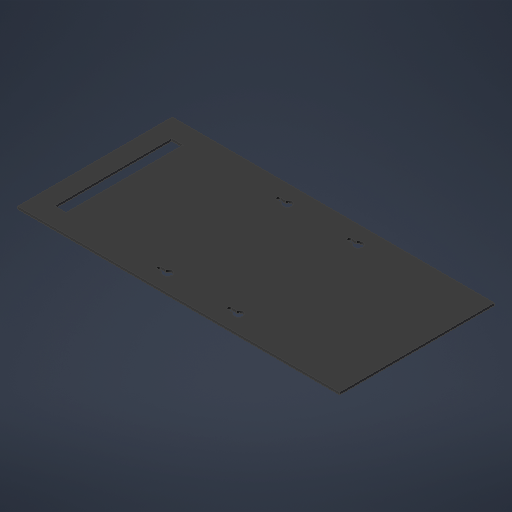
# Autodesk Inventor part: CoverImpresoraTermica
Saved by Autodesk Inventor 2026.1 (Build 301233020, 233B)
## iProperties
Created: 2025-11-04
Part Number: CoverImpresoraTermica
Material: Generic
Document SubType Name: Modeling
Designer: Tito Luyo Murata
Density: 1 g/cm^3
Appearance: Default
Author: Tito Luyo Murata
Autodesk Inventor part; units mm, degrees
ref_plane "YZ Plane" through (0, 0, 0) normal (1, 0, 0) x (0, 1, 0)
ref_plane "XZ Plane" through (0, 0, 0) normal (0, 1, 0) x (-1, 0, 0)
ref_plane "XY Plane" through (0, 0, 0) normal (0, 0, 1) x (1, 0, 0)
sketch "Sketch1" plane through (0, 0, 0) normal (0, 1, 0) x (-1, 0, 0)
  line L0 (0, 0) -> (250, 0)
  line L1 (250, 0) -> (250, -120)
  line L2 (250, -120) -> (0, -120)
  line L3 (0, -120) -> (0, 0)
  arc A0 (95.1623, -105) -> (95.1623, -108) centre (92, -106.5) ccw
  line L4 (236, -14.5) -> (227, -14.5)
  line L5 (227, -14.5) -> (227, -105.5)
  line L6 (227, -105.5) -> (236, -105.5)
  line L7 (236, -105.5) -> (236, -14.5)
  line L8 (95.1623, -105) -> (99, -105)
  line L9 (99, -108) -> (95.1623, -108)
  arc A1 (99, -108) -> (99, -105) centre (99, -106.5) ccw
  arc A2 (99, -15) -> (99, -12) centre (99, -13.5) ccw
  line L10 (95.1623, -12) -> (99, -12)
  arc A3 (95.1623, -12) -> (95.1623, -15) centre (92, -13.5) ccw
  line L11 (99, -15) -> (95.1623, -15)
  arc A4 (154, -108) -> (154, -105) centre (154, -106.5) ccw
  line L12 (150.1623, -105) -> (154, -105)
  arc A5 (150.1623, -105) -> (150.1623, -108) centre (147, -106.5) ccw
  line L13 (154, -108) -> (150.1623, -108)
  arc A6 (154, -15) -> (154, -12) centre (154, -13.5) ccw
  line L14 (150.1623, -12) -> (154, -12)
  arc A7 (150.1623, -12) -> (150.1623, -15) centre (147, -13.5) ccw
  line L15 (154, -15) -> (150.1623, -15)
  point P0 (0, -60)
  point P1 (250, -60)
  dimension "d0" = 250
  dimension "d1" = 120
  dimension "d4" = 7
  dimension "d5" = 92
  dimension "d14" = 9
  dimension "d15" = 91
  dimension "d16" = 45.5
  dimension "d28" = 46.5
  dimension "d31" = 3
  dimension "d32" = 7
  dimension "d33" = 1.5
  dimension "d34" = 3
  dimension "d35" = 7
  dimension "d38" = 93
  dimension "d41" = 55
  dimension "d44" = 80
  constraints: 32 end point, 16 point on circle, 8 centre point, 5 parallel, 4 horizontal, 2 midpoint, 2 perpendicular, 1 vertical, 30 other
  measures "d0" distance of L1.end L2.end
  measures "d1" distance of L0.end L1.end
  measures "d4" diameter of A0
  measures "d5" distance from line of L3 A0.centre
  measures "d14" distance between parallel lines of L5 L7
  measures "d15" distance between parallel lines of L6 L4
  measures "d16" distance from line of point (250, -60) L4
  measures "d28" vertical distance of point (0, -60) A0.centre
  measures "d31" distance between parallel lines of L9 L8
  measures "d32" horizontal distance of A0.centre L8.end
  measures "d33" vertical distance of A0.centre L8.end
  measures "d34" diameter of A1
  measures "d35" distance of A0.centre A1.centre
  measures "d38" distance of A1.centre A2.centre
  measures "d41" distance of A1.centre A4.centre
  measures "d44" distance from line of A5.centre L5
extrude "Extrusion1" add sketch "Sketch1" along normal blind 2
equation "\"d4\" = hueco_diam"
equation "\"d5\" = primer_hueco_dist"
equation "\"d14\" = boca_alto"
equation "\"d15\" = boca_ancho"
equation "\"d16\" = 0.5 * boca_ancho"
equation "\"d28\" = 0.5 * huecos_horiz_dist"
equation "\"d31\" = hueco_ranura_ancho"
equation "\"d32\" = -0.5 * hueco_diam + hueco_ranura_largo - 0.5 * hueco_ranura_ancho"
equation "\"d33\" = 0.5 * hueco_ranura_ancho"
equation "\"d34\" = hueco_ranura_ancho"
equation "\"d35\" = -0.5 * hueco_diam + hueco_ranura_largo - 0.5 * hueco_ranura_ancho"
equation "\"d38\" = huecos_horiz_dist"
equation "\"d41\" = hueco_vertical_dist"
equation "\"d44\" = boca_vertical_dist"
equation "\"hueco_diam\" = 7"
equation "\"primer_hueco_dist\" = 92"
equation "\"huecos_horiz_dist\" = 93"
equation "\"hueco_ranura_ancho\" = 3"
equation "\"hueco_ranura_largo\" = 12"
equation "\"hueco_vertical_dist\" = 55"
equation "\"boca_ancho\" = 91"
equation "\"boca_alto\" = 9"
equation "\"boca_vertical_dist\" = 80"
body "Solid1"
